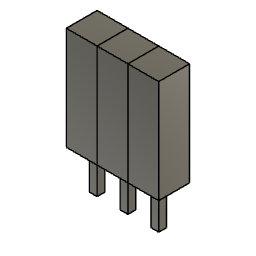
Portable EC device (Autodesk Fusion 360 archive; units mm, degrees)
design "Female Headers"
Autodesk Fusion 360 part; units mm, degrees
sketch "Sketch2" plane through (0, 0, 0) normal (1, 0, 0) x (0, 1, 0)
  line L0 (0, 0) -> (1.27, 0) construction
  line L1 (1.27, 0) -> (-1.27, 0)
  line L2 (-1.27, 0) -> (-1.27, 8.5)
  line L3 (-1.27, 8.5) -> (1.27, 8.5)
  line L4 (1.27, 8.5) -> (1.27, 0)
  line L5 (0, 0) -> (-0.32, 0) construction
  line L6 (-0.32, 0) -> (0.32, 0)
  line L7 (0.32, 0) -> (0.32, -3.2)
  line L8 (0.32, -3.2) -> (-0.32, -3.2)
  line L9 (-0.32, -3.2) -> (-0.32, 0)
  dimension "d1" = 1.27
  dimension "d2" = 2.54
  dimension "d3" = 8.5
  dimension "d4" = 0.32
  dimension "d5" = 0.64
  dimension "d6" = 3.2
  constraint coincident L0.start L5.start
  constraint horizontal L0
  constraint horizontal L1
  constraint vertical L2
  constraint horizontal L3
  constraint vertical L4
  constraint parallel L1 L5
  constraint horizontal L6
  constraint vertical L7
  constraint horizontal L8
  constraint vertical L9
  measures "d1" distance of L0.start L0.end
  measures "d2" distance of L0.end L1.end
  measures "d3" distance of L0.end L3.end
  measures "d4" distance of L0.start L5.end
  measures "d5" distance of L5.end L6.end
  measures "d6" distance of L5.end L8.end
extrude "Extrude1" add sketch "Sketch2" along normal mid plane 2.54 contours L1 L2 L3 L4 L6 makes body 1
extrude "Extrude2" add sketch "Sketch2" along normal mid plane 0.64 contours L1 L6 L7 L8 L9 bodies 1
copy_body "CopyPasteBodies1" bodies 1 makes body 2
move_body "Move1" bodies 2 to x (1, 0, 0) y (0, 1, 0) z (0, 0, 1) at (2.54, 0, 0)
copy_body "CopyPasteBodies2" bodies 2 makes body 3
move_body "Move2" bodies 3 to x (1, 0, 0) y (0, 1, 0) z (0, 0, 1) at (2.54, 0, 0)

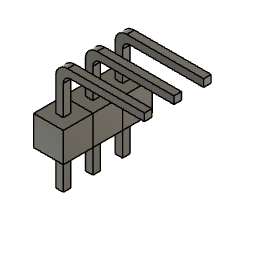
design "Right Angle Headers"
Autodesk Fusion 360 part; units mm, degrees
sketch "Sketch1" plane through (0, 0, 0) normal (0, 1, 0) x (1, 0, 0)
  line L0 (0, 0) -> (0.32, 0) construction
  line L1 (0.32, 0) -> (-0.32, 0)
  line L2 (-0.32, 0) -> (-0.32, -8.36)
  line L3 (0.32, -8.08) -> (0.32, 0)
  line L4 (0.68, -9.36) -> (7.27, -9.36)
  line L5 (7.27, -9.36) -> (7.27, -8.72)
  line L6 (7.27, -8.72) -> (0.96, -8.72)
  arc A0 (-0.32, -8.36) -> (0.68, -9.36) centre (0.68, -8.36) ccw
  arc A1 (0.32, -8.08) -> (0.96, -8.72) centre (0.96, -8.08) ccw
  dimension "d1" = 0.32
  dimension "d2" = 0.64
  dimension "d6" = 1
  dimension "d7" = 0.64
  constraint coincident L0.start origin
  constraint horizontal L0
  constraint horizontal L1
  constraint vertical L2
  constraint vertical L3
  constraint horizontal L4
  constraint vertical L5
  constraint horizontal L6
  constraint tangent L6 A1
  constraint tangent L3 A1
  measures "d1" distance of L0.start L0.end
  measures "d2" distance of L0.end L1.end
  measures "d6" radius of A0
  measures "d7" radius of A1
extrude "Extrude1" add sketch "Sketch1" along normal blind 0.32 and the other way blind 0.32 makes body 1
sketch "Sketch2" plane through (0, 0, 0) normal (0, 1, 0) x (-1, 0, 0)
  line L0 (-0.32, 0) -> (0.32, 0)
  line L1 (0.32, 0) -> (0.32, 8.08)
  arc A0 (0.96, 8.72) -> (0.32, 8.08) centre (0.96, 8.08) ccw
  line L2 (0.96, 8.72) -> (7.27, 8.72)
  line L3 (7.27, 8.72) -> (7.27, 9.36)
  line L4 (7.27, 9.36) -> (0.68, 9.36)
  arc A1 (0.68, 9.36) -> (-0.32, 8.36) centre (0.68, 8.36) ccw
  line L5 (-0.32, 8.36) -> (-0.32, 0)
  line L6 (0, 0) -> (0, 3) construction
  line L7 (0, 3) -> (0, 4.27) construction
  line L8 (1.27, 3) -> (-1.27, 3)
  line L9 (-1.27, 3) -> (-1.27, 5.54)
  line L10 (-1.27, 5.54) -> (1.27, 5.54)
  line L11 (1.27, 5.54) -> (1.27, 3)
  line L12 (1.27, 3) -> (-1.27, 5.54) construction
  line L13 (-1.27, 3) -> (1.27, 5.54) construction
  point P0 (0, 4.27)
  dimension "d12" = 3
  dimension "d13" = 1.27
  dimension "d14" = 2.54
  dimension "d15" = 2.54
  constraint coincident L6.start origin
  constraint perpendicular L0 L6
  constraint parallel L6 L7
  constraint horizontal L8
  constraint perpendicular L8 L9
  constraint parallel L8 L10
  constraint parallel L9 L11
  constraint coincident L12 P0
  constraint coincident L13 P0
  constraint coincident P0 L7.end
  measures "d12" distance of L6.start L6.end
  measures "d13" distance of L6.end P0
  measures "d14" distance of L9.end L10.end
  measures "d15" distance of L8.end L9.end
extrude "Extrude2" add sketch "Sketch2" along normal mid plane 2.54 contours L5 L8 L9 L10 | L1 L5 L8 L10 | L1 L8 L10 L11 bodies 1
copy_body "CopyPasteBodies1" bodies 1 makes body 2
move_body "Move1" bodies 2 to x (1, 0, 0) y (0, 1, 0) z (0, 0, 1) at (0, 2.54, 0)
copy_body "CopyPasteBodies2" bodies 2 makes body 3
move_body "Move2" bodies 3 to x (1, 0, 0) y (0, 1, 0) z (0, 0, 1) at (0, 2.54, 0)
equation "d1 = ( 0.64 / 2 ) * 1 mm"
equation "d13 = ( 2.54 / 2 ) * 1 mm"
